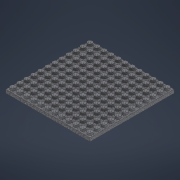
# Autodesk Inventor part: 110033226_ipt_05_房子底座
Saved by Autodesk Inventor 2022 (Build 260153000, 153)
## iProperties
Created: 2022-06-22
Part Number: 110033226_ipt_05_房子底座
Material: 一般
Document SubType Name: Modeling
Designer: User
Density: 1 g/cm^3
Appearance: 預設
Author: User
Autodesk Inventor part; units mm, degrees
ref_plane "YZ Plane" through (0, 0, 0) normal (1, 0, 0) x (0, 1, 0)
ref_plane "XZ Plane" through (0, 0, 0) normal (0, 1, 0) x (-1, 0, 0)
ref_plane "XY Plane" through (0, 0, 0) normal (0, 0, 1) x (1, 0, 0)
sketch "草圖1" plane through (0, 0, 0) normal (0, 1, 0) x (-1, 0, 0)
  line L0 (30, 30) -> (-30, 30)
  line L1 (-30, 30) -> (-30, -30)
  line L2 (-30, -30) -> (30, -30)
  line L3 (30, -30) -> (30, 30)
  point P0 (0, 0)
  point P1 (0, 30)
  point P2 (30, 0)
  dimension "d0" = 60
  dimension "d1" = 60
  constraints: 8 end point, 2 midpoint, 2 parallel, 1 horizontal, 1 horizontal alignment, 1 perpendicular, 1 vertical alignment
  measures "d0" distance of L2.end L1.end
  measures "d1" distance of L1.end L0.end
extrude "擠出1" add sketch "草圖1" along normal blind 2.5
sketch "草圖2" plane through (0, 2.5, 0) normal (0, 1, 0) x (1, 0, 0)
  line L0 (30, -30) -> (30, 30) projected
  line L1 (30, 30) -> (-30, 30) projected
  line L2 (-30, 30) -> (-30, -30) projected
  line L3 (-30, -30) -> (30, -30) projected
  circle A0 centre (27.5, -27.5) radius 1.7
  point P0 (0, 0)
  dimension "d4" = 3.4
  dimension "d5" = 2.5
  dimension "d6" = 2.5
  constraints: 1 centre point
  measures "d4" diameter of A0
  measures "d5" distance from line of L0 A0.centre
  measures "d6" distance from line of L3 A0.centre
extrude "擠出2" add sketch "草圖2" along normal blind 1.5 contours A0
pattern_linear "矩形陣列1" count 12 spacing 5 along (0, 0, -1) count 12 spacing 5 along (-1, 0, 0) of "擠出2"
sketch "草圖3" plane through (0, 0, 0) normal (0, -1, 0) x (1, 0, 0)
  line L0 (-30, 30) -> (30, 30) projected
  line L1 (30, 30) -> (30, -30) projected
  line L2 (30, -30) -> (-30, -30) projected
  line L3 (-30, -30) -> (-30, 30) projected
  circle A0 centre (-27.5, 27.5) radius 1.7 projected
  point P0 (0, 0)
extrude "擠出3" cut sketch "草圖3" against normal blind 1.5 contours A0
pattern_linear "矩形陣列2" count 12 spacing 5 along (1, 0, 0) count 12 spacing 5 along (0, 0, -1) of "擠出3"
